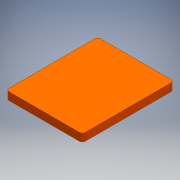
# Autodesk Inventor part: sampleMount
Saved by Autodesk Inventor 2016 (Build 200138000, 138)
## iProperties
Created: 2016-11-09
Part Number: sampleMount
Material: Generic
Document SubType Name: Modeling
Designer: sims01
Density: 1 g/cm^3
Appearance: Default
Author: sims01
Autodesk Inventor part; units mm, degrees
ref_plane "YZ Plane" through (0, 0, 0) normal (1, 0, 0) x (0, 1, 0)
ref_plane "XZ Plane" through (0, 0, 0) normal (0, 1, 0) x (-1, 0, 0)
ref_plane "XY Plane" through (0, 0, 0) normal (0, 0, 1) x (1, 0, 0)
sketch "Sketch1" plane through (0, 0, 0) normal (0, 0, 1) x (1, 0, 0)
  line L0 (-23, 30) -> (23, 30)
  line L1 (25, 28) -> (25, -28)
  line L2 (23, -30) -> (-23, -30)
  line L3 (-25, -28) -> (-25, 28)
  arc A0 (-23, 30) -> (-25, 28) centre (-23, 28) ccw
  arc A1 (-25, -28) -> (-23, -30) centre (-23, -28) ccw
  arc A2 (23, -30) -> (25, -28) centre (23, -28) ccw
  arc A3 (25, 28) -> (23, 30) centre (23, 28) ccw
  point P0 (0, 0)
  point P1 (-25, 30)
  point P2 (25, -30)
  point P3 (25, 30)
  dimension "d0" = 60
  dimension "d1" = 50
  dimension "d2" = 30
  dimension "d3" = 25
  dimension "d4" = 2
  constraints: 8 end point, 8 point on circle, 8 tangent, 6 point on line, 4 centre point, 3 equal radius, 2 parallel, 1 horizontal, 1 perpendicular
  measures "d0" distance of point (25, 30) point (25, -30)
  measures "d1" distance of point (-25, 30) point (25, 30)
  measures "d2" distance from line of point (0, 0) L0
  measures "d3" distance from line of point (0, 0) L1
  measures "d4" radius of A0
extrude "base" add sketch "Sketch1" along normal blind 5
sketch "Sketch3" plane through (0, 0, 0) normal (0, 0, -1) x (-1, 0, 0)
  circle A0 centre (0, -15) radius 1.325
  circle A1 centre (15, 0) radius 1.325
  circle A2 centre (0, 15) radius 1.325
  circle A3 centre (-15, 0) radius 1.325
  circle A4 centre (0, 0) radius 1.325
  dimension "d7" = 2.65
  dimension "d8" = 2.65
  dimension "d9" = 2.65
  dimension "d10" = 2.65
  dimension "d11" = 2.65
  dimension "d12" = 15
  dimension "d13" = 15
  dimension "d14" = 15
  dimension "d15" = 15
  constraints: 5 centre point, 2 coincident, 2 horizontal alignment, 2 vertical alignment
  measures "d7" diameter of A0
  measures "d8" diameter of A1
  measures "d9" diameter of A4
  measures "d10" diameter of A3
  measures "d11" diameter of A2
  measures "d12" distance of point (0, 0) A0.centre
  measures "d13" distance of A3.centre point (0, 0)
  measures "d14" distance of A2.centre point (0, 0)
  measures "d15" distance of A1.centre point (0, 0)
extrude "magnetMount" cut sketch "Sketch3" against normal blind 2
equation "\"d2\" = 0.5 * d0"
equation "\"d3\" = 0.5 * d1"
equation "\"d8\" = d7"
equation "\"d9\" = d7"
equation "\"d10\" = d7"
equation "\"d11\" = d7"
equation "\"d13\" = d12"
equation "\"d14\" = d12"
equation "\"d15\" = d13"
body "Solid1"
